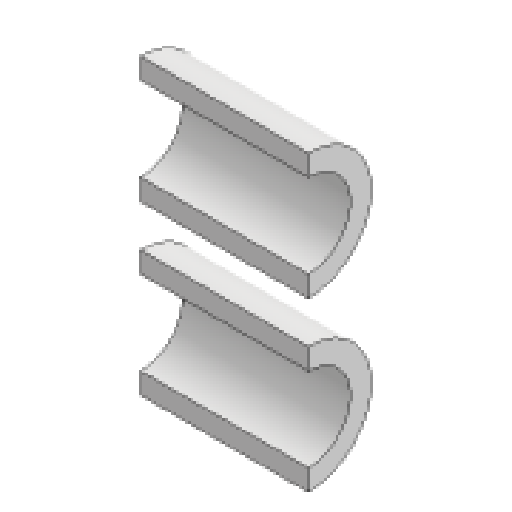
# Autodesk Inventor part: Carbon4BarCrossbarclamping hub
Saved by Autodesk Inventor 2023 (Build 270158000, 158)
## iProperties
Created: 2022-10-29
Part Number: Carbon4BarCrossbarclamping hub
Material: Generic
Document SubType Name: Modeling
Designer: deli
Density: 1 g/cm^3
Appearance: Default
Author: deli
Autodesk Inventor part; units mm, degrees
ref_plane "YZ Plane" through (0, 0, 0) normal (1, 0, 0) x (0, 1, 0)
ref_plane "XZ Plane" through (0, 0, 0) normal (0, 1, 0) x (-1, 0, 0)
ref_plane "XY Plane" through (0, 0, 0) normal (0, 0, 1) x (1, 0, 0)
sketch "Sketch1" plane through (0, 0, 0) normal (1, 0, 0) x (0, 1, 0)
  circle A0 centre (6.7777, 53.2132) radius 4
  circle A1 centre (-9.2223, 53.2132) radius 4
  line L0 (12.7777, 53.2132) -> (-15.2223, 53.2132)
  circle A2 centre (6.7777, 53.2132) radius 6
  circle A3 centre (-9.2223, 53.2132) radius 6
  line L1 (6.7777, 47.2132) -> (-9.2223, 47.2132)
  point P0 (0, 0)
  point P1 (-3.2223, 53.2132)
  point P2 (-5.2223, 53.2132)
  point P3 (-13.2223, 53.2132)
  point P4 (0.7777, 53.2132)
  point P5 (10.7777, 53.2132)
  point P6 (2.7777, 53.2132)
  dimension "d0" = 8
  dimension "d2" = 2
  dimension "d4" = 16
  constraints: 4 centre point, 4 end point, 4 point on circle, 2 coincident, 2 equal radius, 2 horizontal, 2 point on line
  measures "d0" diameter of A0
  measures "d2" radial gap between concentric circles of A0 A2
  measures "d4" distance of A1.centre A0.centre
extrude "Extrusion1" add sketch "Sketch1" along normal blind 16 contours L0 A2 A0 | A2 L1 A3 L0 | A3 L0 A1 picked at (1.4945, 52.7682) picked at (-14.5055, 52.7682)
sketch "Sketch3" plane through (0, 0, 0) normal (-1, 0, 0) x (0, 0, 1)
  arc A0 (53.2132, 12.7777) -> (47.2132, 6.7777) centre (53.2132, 6.7777) ccw projected
  arc A1 (47.2132, -9.2223) -> (53.2132, -15.2223) centre (53.2132, -9.2223) ccw projected
  line L0 (47.2132, -9.2223) -> (47.2132, 6.7777) projected
  line L1 (53.2132, 2.7777) -> (53.2132, -5.2223) construction
  arc A2 (59.2132, 6.7777) -> (53.2132, 12.7777) centre (53.2132, 6.7777) ccw
  arc A3 (53.2132, -15.2223) -> (59.2132, -9.2223) centre (53.2132, -9.2223) ccw
  line L2 (59.2132, -9.2223) -> (59.2132, 6.7777)
  point P0 (0, 0)
  constraints: 4 point on circle, 2 centre point, 2 end point, 2 symmetric about line, 2 other
extrude "Extrusion2" add sketch "Sketch3" along normal blind 2
sketch "Sketch5" plane through (-2, 0, 0) normal (-1, 0, 0) x (0, 0, 1)
  circle A0 centre (53.2132, -1.2223) radius 4
  line L0 (47.2132, -9.2223) -> (47.2132, 6.7777) construction
  arc A1 (53.2132, -15.2223) -> (59.2132, -9.2223) centre (53.2132, -9.2223) ccw construction
  line L1 (47.2132, 6.7777) -> (59.2132, -9.2223) construction
  point P0 (0, 0)
  dimension "d9" = 8
  constraints: 2 end point, 1 centre point, 1 coincident, 1 midpoint
  measures "d9" diameter of A0
extrude "Extrusion3" add sketch "Sketch5" along normal blind 23.5
sketch "Sketch6" plane through (-25.5, -1.2223, 53.2132) normal (-1, 0, 0) x (0, 0, 1)
  line L0 (0, 4) -> (0, -4) projected
  line L1 (-4.0415, 0) -> (-2.0207, 3.5)
  line L2 (-2.0207, 3.5) -> (2.0207, 3.5)
  line L3 (2.0207, 3.5) -> (4.0415, 0)
  line L4 (4.0415, 0) -> (2.0207, -3.5)
  line L5 (2.0207, -3.5) -> (-2.0207, -3.5)
  line L6 (-2.0207, -3.5) -> (-4.0415, 0)
  circle A0 centre (0, 0) radius 4 projected
  point P0 (-53.2132, 1.2223)
  point P1 (0, 0)
  point P2 (-3.9993, -0.0729)
  point P3 (-2.0628, -3.4271)
  point P4 (1.9365, -3.5)
  point P5 (-1.9365, -3.5)
  point P6 (2.0628, -3.4271)
  point P7 (3.9993, -0.0729)
  point P8 (3.9993, 0.0729)
  point P9 (2.0628, 3.4271)
  point P10 (-1.9365, 3.5)
  point P11 (1.9365, 3.5)
  point P12 (-2.0628, 3.4271)
  point P13 (-3.9993, 0.0729)
  dimension "d12" = 7
  constraints: 12 end point, 1 horizontal, 1 midpoint, 13 other
  measures "d12" distance between parallel lines of L5 L2
extrude "Extrusion4" cut sketch "Sketch6" against normal blind 10.5 contours A0 L2 L0 | L0 L2 A0 | L5 A0 L0 | L0 A0 L5 | A0 L3 | L1 A0 | L4 A0 | A0 L6
sketch "Sketch7" plane through (16, -5.2223, 53.2132) normal (0, 0, 1) x (1, 0, 0)
  circle A0 centre (-8, 4) radius 2
  line L0 (-16, 8) -> (0, 8) construction
  line L1 (-16, 8) -> (0, 0) construction
  point P0 (-16, 5.2223)
  point P1 (-8, 4)
  dimension "d15" = 4
  constraints: 2 end point, 1 centre point, 1 coincident, 1 midpoint
  measures "d15" diameter of A0
extrude "Extrusion5" cut sketch "Sketch7" against normal blind 10.5
thread "Thread1" size "M4x0.7" class "6H" standard "ANSI Metric M Profile" full length
body "Solid1"
